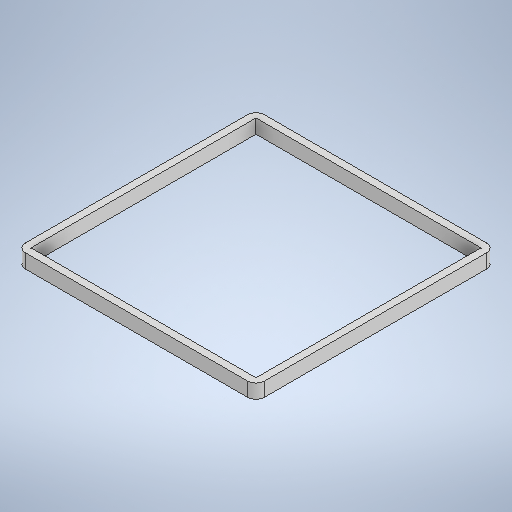
# Autodesk Inventor part: こたつの足_試作
Saved by Autodesk Inventor 2025 (Build 290162000, 162)
## iProperties
Created: 2025-11-12
Part Number: こたつの足_試作
Material: 一般
Document SubType Name: Modeling
Designer: mahhy
Density: 1 g/cm^3
Appearance: 既定
Author: mahhy
Autodesk Inventor part; units mm, degrees
ref_plane "YZ Plane" through (0, 0, 0) normal (1, 0, 0) x (0, 1, 0)
ref_plane "XZ Plane" through (0, 0, 0) normal (0, 1, 0) x (-1, 0, 0)
ref_plane "XY Plane" through (0, 0, 0) normal (0, 0, 1) x (1, 0, 0)
sketch "スケッチ1" plane through (0, 0, 0) normal (0, 1, 0) x (-1, 0, 0)
  line L0 (0, 0) -> (85, 0)
  line L1 (85, 0) -> (85, -85)
  line L2 (85, -85) -> (0, -85)
  line L3 (0, -85) -> (0, 0)
  line L4 (82.5, -2.5) -> (2.5, -2.5)
  line L5 (2.5, -2.5) -> (2.5, -82.5)
  line L6 (2.5, -82.5) -> (82.5, -82.5)
  line L7 (82.5, -82.5) -> (82.5, -2.5)
  point P0 (42.5, -2.5)
  point P1 (42.5, 0)
  point P2 (82.5, -42.5)
  point P3 (85, -42.5)
  dimension "d0" = 85
  dimension "d1" = 85
  dimension "d2" = 80
  dimension "d3" = 80
  constraints: 16 end point, 4 midpoint, 4 parallel, 2 horizontal, 2 perpendicular, 1 horizontal alignment, 1 vertical alignment
  measures "d0" distance of L1.end L2.end
  measures "d1" distance of L0.end L1.end
  measures "d2" distance of L6.end L5.end
  measures "d3" distance of L5.end L4.end
extrude "押し出し1" add sketch "スケッチ1" along normal blind 5
fillet "フィレット1" radius 3 4 edges at (0, 2.5, 0) (-85, 2.5, 0) (-85, 2.5, -85) (0, 2.5, -85)
